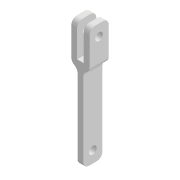
# Autodesk Inventor part: brazo_servo
Saved by Autodesk Inventor 2022 (Build 260153000, 153)
## iProperties
Created: 2022-11-01
Part Number: brazo_servo
Material: Genérico
Document SubType Name: Modeling
Designer: Jorge
Density: 1 g/cm^3
Appearance: Valor por defecto
Author: Jorge
Autodesk Inventor part; units mm, degrees
ref_plane "YZ Plane" through (0, 0, 0) normal (1, 0, 0) x (0, 1, 0)
ref_plane "XZ Plane" through (0, 0, 0) normal (0, 1, 0) x (-1, 0, 0)
ref_plane "XY Plane" through (0, 0, 0) normal (0, 0, 1) x (1, 0, 0)
sketch "Boceto1" plane through (0, 0, 0) normal (0, 0, 1) x (1, 0, 0)
  line L0 (0, 45) -> (-3.25, 45)
  line L1 (-3.25, 45) -> (-3.25, 65)
  line L2 (-3.25, 65) -> (-0.25, 65)
  line L3 (-0.25, 65) -> (-0.25, 48)
  line L4 (-0.25, 48) -> (3.25, 48)
  line L5 (3.25, 48) -> (3.25, 65)
  line L6 (3.25, 65) -> (6.25, 65)
  line L7 (6.25, 65) -> (6.25, 45)
  line L8 (6.25, 45) -> (3, 45)
  line L9 (3, 0) -> (0, 0)
  line L10 (1.5, 0) -> (1.5, 40) construction
  line L11 (0, 0) -> (0, 15)
  line L12 (0, 15) -> (0, 45)
  line L13 (3, 45) -> (3, 15)
  line L14 (3, 15) -> (3, 0)
  dimension "d1" = 3
  dimension "d4" = 3
  dimension "d5" = 3.5
  dimension "d6" = 9.5
  dimension "d8" = 4.75
  dimension "d9" = 20
  dimension "d20" = 3
  dimension "d27" = 65
  constraints: 30 end point, 12 perpendicular, 4 point on line, 3 vertical, 1 midpoint
  measures "d1" distance of L1.end L2.end
  measures "d4" distance between parallel lines of L7 L5
  measures "d5" distance between parallel lines of L5 L3
  measures "d6" distance between parallel lines of L7 L1
  measures "d8" distance between parallel lines of L10 L1
  measures "d9" distance of L0.end L1.end
  measures "d20" distance between parallel lines of L8 L4
  measures "d27" distance between parallel lines of L9 L2
extrude "Extrusión1" add sketch "Boceto1" along normal blind 10
sketch "Boceto2" plane through (6.25, 45, 0) normal (1, 0, 0) x (0, 0, -1)
  line L0 (0, 3) -> (-10, 3) construction
  line L1 (0, 0) -> (0, 20) construction
  line L2 (0, 20) -> (-10, 20) construction
  line L3 (-10, 0) -> (-10, 20) construction
  line L4 (0, 0) -> (-10, 0) construction
  line L5 (-10, 0) -> (-10, 20) construction
  line L6 (-10, 20) -> (-10, 3) construction
  line L7 (-10, 14) -> (0, 14) construction
  circle A0 centre (-5, 14) radius 2
  point P0 (0, -45)
  dimension "d15" = 4
  dimension "d16" = 6
  constraints: 2 end point, 2 point on line, 1 centre point, 1 midpoint, 1 perpendicular
  measures "d15" diameter of A0
  measures "d16" distance between parallel lines of L2 L7
extrude "Extrusión2" cut sketch "Boceto2" against normal through all
fillet "Empalme1" radius 3 10 edges at (-1.75, 65, 10) (-1.75, 65, 0) (4.75, 65, 0) (4.75, 65, 10) (0, 45, 5) (3, 45, 5) (6.25, 45, 5) (-3.25, 45, 5) (1.5, 0, 10) (1.5, 0, 0)
sketch "Boceto4" plane through (3, 3, 0) normal (1, 0, 0) x (0, 0, -1)
  arc A0 (-10, 0) -> (-7, -3) centre (-7, 0) ccw construction
  line L0 (0, 0) -> (0, 39) construction
  line L1 (-10, 39) -> (0, 39) construction
  line L2 (-10, 0) -> (-10, 39) construction
  line L3 (-3, -3) -> (-7, -3) projected
  line L4 (-3, -3) -> (-7, -3) construction
  line L5 (-5, -3) -> (-5, 39) construction
  line L6 (0, 39) -> (-10, 39) construction
  circle A1 centre (-5, 3) radius 2
  arc A2 (-3, -3) -> (0, 0) centre (-3, 0) ccw projected
  point P0 (0, -3)
  dimension "d28" = 4
  dimension "d29" = 6
  constraints: 2 end point, 2 midpoint, 1 centre point, 1 point on line
  measures "d28" diameter of A1
  measures "d29" distance from line of L3 A1.centre
extrude "Extrusión3" cut sketch "Boceto4" against normal blind 10
equation "\"d8\" = 0.5 * d6"
